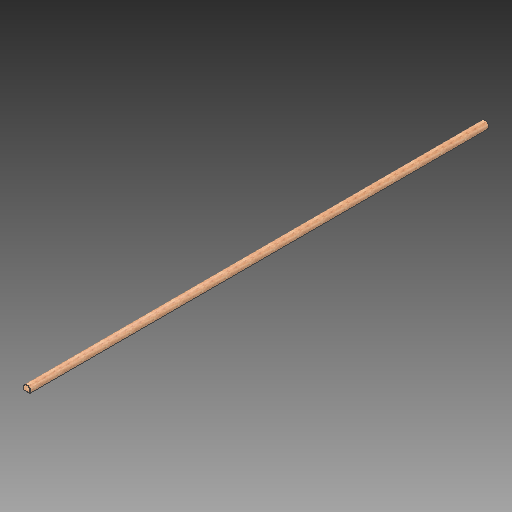
# Autodesk Inventor part: træhåndfang
Saved by Autodesk Inventor 2018 (Build 220112000, 112)
## iProperties
Created: 2019-09-28
Part Number: træhåndfang
Material: Wood (Birch)
Document SubType Name: Modeling
Designer: loppen
Density: 0.55 g/cm^3
Appearance: Birch - Natural Polished
Mass: 11829.5 g
Surface Area: 12525.9 cm^2
Volume: 21508.1 cm^3
Author: loppen
Autodesk Inventor part; units mm, degrees
ref_plane "YZ Plane" through (0, 0, 0) normal (1, 0, 0) x (0, 1, 0)
ref_plane "XZ Plane" through (0, 0, 0) normal (0, 1, 0) x (-1, 0, 0)
ref_plane "XY Plane" through (0, 0, 0) normal (0, 0, 1) x (1, 0, 0)
sketch "Sketch1" plane through (0, 0, 0) normal (0, 0, 1) x (1, 0, 0)
  circle A0 centre (0, 0) radius 40
  line L0 (-56, 0) -> (56, 0) projected
  line L1 (-4, -26.4575) -> (-4, -20.4575)
  line L2 (-4, -20.4575) -> (4, -20.4575)
  line L3 (4, -20.4575) -> (4, -26.4575)
  line L4 (-30, -26.4575) -> (-4, -26.4575)
  line L5 (4, -26.4575) -> (30, -26.4575)
  dimension "d0" = 80
  dimension "d1" = 60
  dimension "d2" = 6
  dimension "d3" = 26
  dimension "d4" = 8
  constraints: 10 end point, 5 perpendicular, 2 parallel, 2 point on circle, 1 centre point, 1 coincident, 1 collinear
  measures "d0" diameter of A0
  measures "d1" distance of L4.start L5.end
  measures "d2" distance of L2.end L3.end
  measures "d3" distance from line of L4.start L1
  measures "d4" distance of L1.end L2.end
extrude "Extrusion1" add sketch "Sketch1" along normal blind 4871.551 contours A0 L0 L5 L3 L2 L1 L4 | A0 L0
fillet "Fillet1" radius 4 6 edges at (0, 40, 0) (-17, -26.4575, 0) (17, -26.4575, 0) (0, 40, 4871.551) (17, -26.4575, 4871.551) (-17, -26.4575, 4871.551)
equation "\"d3\" = -0.5 * d4 + 0.5 * d1"
body "Solid1"
